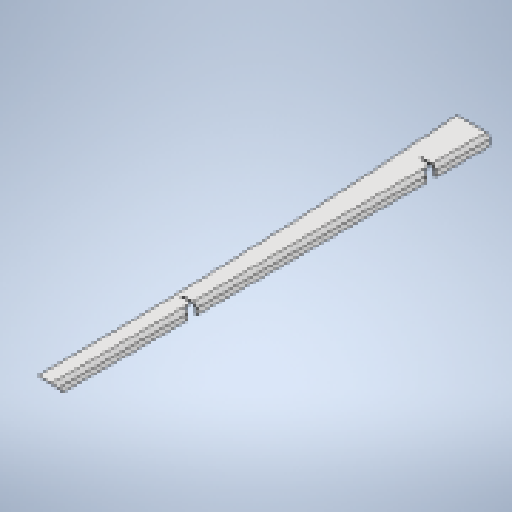
# Autodesk Inventor part: MSC 312 RIB HIP
Saved by Autodesk Inventor 2025.1 (Build 291241020, 241B)
## iProperties
Created: 2024-04-28
Part Number: MSC 312 RIB HIP
Material: Stainless Steel
Description: DIE16(5)|\ 90°|corrY -___°|X_____|bom___
Document SubType Name: Sheet Metal
Designer: pokla
Stock Number: MSC 315 шпангоут борт
Density: 8 g/cm^3
Flat Pattern Width: 91.0953 cm
Flat Pattern Length: 8.39274 cm
Flat Pattern Area: 764.54 cm^2
Sheet Metal Rule: AISI304 3mm Die 32
Sheet Metal Width: 910.953 mm
Sheet Metal Length: 83.927 mm
Sheet Metal Area: 76453.964 mm^2
Appearance: Default
Mass: 990.281 g
Surface Area: 1284.73 cm^2
Volume: 123.785 cm^3
БОРТ_стрингер_3_высота: 62,000 mm
БОРТ_стрингер_4_высота: 39,000 mm
БОРТ_стрингер_5_высота: 39,000 mm
БОРТ_стрингер_6_высота: 62,000 mm
РЕБРА_глубина_паза: 28.000 mm
РЕБРА_вырез_на_полке: 5,000 mm
РЕБРА_полка: 20,000 mm
Author: admin
Autodesk Inventor part; units mm, degrees
ref_plane "YZ Plane" through (0, 0, 0) normal (1, 0, 0) x (0, 1, 0)
ref_plane "XZ Plane" through (0, 0, 0) normal (0, 1, 0) x (-1, 0, 0)
ref_plane "XY Plane" through (0, 0, 0) normal (0, 0, 1) x (1, 0, 0)
sketch "Sketch1" plane through (0, 0, 0) normal (0, 0, 1) x (1, 0, 0)
  arc A0 (-71.9586, -1745.1712) -> (-70, 0) centre (-11089.4751, -860.2193) ccw
  line L0 (0, 0) -> (-70, 0)
  line L1 (0, -117.9106) -> (-61.4296, -117.9106) construction
  line L2 (0, -617.9106) -> (-39.1314, -617.9106) construction
  line L3 (0, -1117.9106) -> (-39.4794, -1117.9106) construction
  line L4 (0, -1617.9106) -> (-62.4758, -1617.9106) construction
  line L5 (-71.9586, -1745.1712) -> (0, -1745.1712)
  line L6 (0, 0) -> (0, -1745.1712)
  line L7 (0, -1735.1712) -> (-10.3553, -1745.1712)
  point P0 (-20, 0)
  dimension "d33" = 50
  dimension "d58" = 500
  dimension "d59" = 500
  dimension "d60" = 500
  dimension "d141" = 1745.171
  dimension "d148" = 70
  dimension "d149" = 11053
  dimension "d150" = 71.959
  dimension "d151" = 136
  dimension "d153" = 10
  measures "d33" distance of L0.end point (-20, 0)
  measures "d58" distance between parallel lines of L2 L1
  measures "d59" distance between parallel lines of L2 L3
  measures "d60" distance between parallel lines of L3 L4
  measures "d141" distance between parallel lines of L0 L5
  measures "d148" distance of L0.start L0.end
  measures "d149" radius of A0
  measures "d151" angle of L5 L7
  measures "d153" distance of L5.end L7.start
extrude "Plate3" add sketch "Sketch1" along normal blind 3 contours A0 L0 L6 L7 L5
sketch "Sketch3" plane through (-3, 0, 3) normal (1, 0, 0) x (0, 1, 0)
  line L0 (-1735.1712, 0) -> (0, 0)
  line L1 (0, 0) -> (0, 20)
  line L2 (0, 20) -> (-1735.1712, 20)
  line L3 (-1735.1712, 20) -> (-1735.1712, 0)
  constraints: 6 end point, 1 horizontal, 1 perpendicular, 1 vertical
edge flange "Flange2" height 20 angle 90 thickness 3 bend radius 5 thickness toward (1, 0, 0) relief round relief width 3 relief depth 1.5 edges at (0, -867.5856, 3) wall of the first edge with corners at (-3, -1735.1712, 3) (-3, 0, 3) (-3, 0, -17) (-3, -1735.1712, -17)
bend "Bend2"
corner "Corner2"
sketch "Sketch5" plane through (0, 0, 0) normal (0, 0, 1) x (1, 0, 0)
  line L0 (-8, -1742.8967) -> (-8, 0) projected
  line L1 (-70, 0) -> (-8, 0) projected
  arc A0 (-71.9586, -1745.1712) -> (-70, 0) centre (-11089.4751, -860.2193) ccw projected
  line L2 (0, 0) -> (0, -1735.1712) projected
  line L3 (0, -114.5) -> (-29, -114.5)
  line L4 (0, -117.5) -> (-3, -117.5) construction
  line L5 (-3, -1735.1712) -> (-3, 0) projected
  line L6 (-29, -114.5) -> (-29, -117.5)
  line L7 (0, -614.5) -> (-39.2067, -614.5) construction
  line L8 (0, -1114.5) -> (-39.4004, -1114.5) construction
  line L9 (0, -1614.5) -> (-62.242, -1614.5) construction
  line L10 (-10.3553, -1745.1712) -> (-71.9586, -1745.1712) projected
  line L11 (0, -114.5) -> (0, -134.5)
  line L12 (-3, -114.5) -> (-3, -117.5) construction
  line L13 (0, -134.5) -> (-3, -134.5)
  line L14 (-29, -114.5) -> (-61.6597, -114.5) construction
  line L15 (-29, -117.5) -> (-61.4573, -117.5) construction
  line L16 (-3, -117.5) -> (-3, -134.5)
  line L17 (-3, -117.5) -> (-29, -117.5)
  line L18 (-3, -134.5) -> (-8, -134.5)
  line L19 (-8, -1742.8967) -> (-10.3553, -1745.1712) projected
  point P0 (0, 0)
  point P1 (845.25, -380.4205)
  point P2 (848, -380.4205)
  point P3 (-29, -116)
  point P4 (850, -410.4205)
  point P5 (-3, -114.5)
  point P6 (-3, -134.5)
  point P7 (-8, -117.5)
  dimension "d69" = 1735.1712
  dimension "d70" = 3
  dimension "d76" = 61.6598
  dimension "d80" = 39.2067
  dimension "d102" = 62.242
  dimension "d104" = 39.4004
  dimension "d106" = 3
  dimension "d107" = 20
  dimension "d108" = 116
  dimension "d112" = 29
  dimension "d142" = 500
  dimension "d143" = 500
  dimension "d144" = 500
  constraints: 28 end point, 13 perpendicular, 10 point on line, 5 point on circle, 2 parallel, 1 horizontal, 1 midpoint
  measures "d69" distance of L2.start L2.end
  measures "d70" distance between parallel lines of L4 L3
  measures "d76" distance of L3.start L14.end
  measures "d80" distance of L7.start L7.end
  measures "d102" distance of L9.start L9.end
  measures "d104" distance of L8.end L8.start
  measures "d106" distance of L13.end L11.end
  measures "d107" distance of L11.end L3.start
  measures "d108" vertical distance of L2.start point (-29, -116)
  measures "d112" distance of L3.end L3.start
  measures "d142" distance between parallel lines of L7 L14
  measures "d143" distance between parallel lines of L7 L8
  measures "d144" distance between parallel lines of L9 L8
extrude "Extrusion2" cut sketch "Sketch5" along normal through all both and the other way through all contours L0 L17 L5 L18 | L17 L6 L3 L0 | L0 L3 L5 L17 | L5 L3 L2 L13
pattern_linear "Rectangular Pattern3" count 4 spacing 500 along (0, -1, 0) of "Extrusion2"
sketch "Sketch6" plane through (0, 0, 0) normal (0, 0, -1) x (-1, 0, 0)
  line L0 (25.1246, -1740.1712) -> (13.1246, -1740.1712) construction
  line L1 (13.1246, -1740.1712) -> (13.1246, -1540.1712) construction
  line L2 (13.1246, -1540.1712) -> (25.1246, -1540.1712) construction
  line L3 (25.1246, -1540.1712) -> (25.1246, -1740.1712) construction
  line L4 (25.1246, -1539.5) -> (25.1246, -1589.5) construction
  line L5 (25.1246, -1589.5) -> (13.1246, -1589.5) construction
  line L6 (13.1246, -1589.5) -> (13.1246, -1539.5) construction
  line L7 (13.1246, -1539.5) -> (25.1246, -1539.5) construction
  line L8 (8, -1614.5) -> (29, -1614.5) projected
  line L9 (25.1246, -1039.5) -> (25.1246, -1089.5) construction
  line L10 (25.1246, -1089.5) -> (13.1246, -1089.5) construction
  line L11 (13.1246, -1089.5) -> (13.1246, -1039.5) construction
  line L12 (13.1246, -1039.5) -> (25.1246, -1039.5) construction
  line L13 (25.1246, -539.5) -> (25.1246, -589.5) construction
  line L14 (25.1246, -589.5) -> (13.1246, -589.5) construction
  line L15 (13.1246, -589.5) -> (13.1246, -539.5) construction
  line L16 (13.1246, -539.5) -> (25.1246, -539.5) construction
  line L17 (25.1246, -39.5) -> (25.1246, -89.5) construction
  line L18 (25.1246, -89.5) -> (13.1246, -89.5) construction
  line L19 (13.1246, -89.5) -> (13.1246, -39.5) construction
  line L20 (13.1246, -39.5) -> (25.1246, -39.5) construction
  line L21 (8, -1114.5) -> (29, -1114.5) projected
  line L22 (8, -614.5) -> (29, -614.5) projected
  line L23 (8, -114.5) -> (29, -114.5) projected
  line L24 (25.1246, -740) -> (13.1246, -740) construction
  line L25 (13.1246, -740) -> (13.1246, -540) construction
  line L26 (13.1246, -540) -> (25.1246, -540) construction
  line L27 (25.1246, -540) -> (25.1246, -740) construction
  point P0 (0, 0)
  point P1 (71.9586, -1745.1712)
  point P2 (4.75, -1840)
  point P3 (-1.1417, -614.8288)
  point P4 (25.1083, -614.8288)
  dimension "d120" = 200
  dimension "d121" = 12
  dimension "d123" = 5
  dimension "d126" = 50
  dimension "d127" = 25
  dimension "d135" = 25
  dimension "d136" = 25
  dimension "d137" = 25
  dimension "d154" = 200
  dimension "d155" = 12
  constraints: 7 equal length, 4 collinear, 13 other
  measures "d120" distance of L0.end L1.end
  measures "d121" distance of L1.end L2.end
  measures "d126" distance of L5.end L6.end
  measures "d127" distance between parallel lines of L8 L5
  measures "d135" distance between parallel lines of L21 L10
  measures "d136" distance between parallel lines of L22 L14
  measures "d137" distance between parallel lines of L23 L18
  measures "d154" distance of L24.end L25.end
  measures "d155" distance of L25.end L26.end
chamfer "Corner Chamfer1" distance 6 angle 45 4 edges at (-8, -1617.5, 1.5) (-8, -1117.5, 1.5) (-8, -617.5, 1.5) (-8, -117.5, 1.5)
mark "Mark2"
sketch "Sketch9" plane through (0, -1614.5, -17) normal (1, 0, 0) x (0, 0, -1)
  line L0 (-17, -130.6712) -> (-20, -130.6712) projected
  line L1 (0, 500) -> (0, 980) projected
  line L2 (-20, -130.6712) -> (0, -130.6712)
  line L3 (0, -130.6712) -> (0, 720.3288)
  line L4 (0, 720.3288) -> (-20, 720.3288)
  line L5 (-20, 720.3288) -> (-20, -130.6712)
  line L6 (0, 720.3288) -> (-20, 703.5468)
  line L7 (-20, 1614.5) -> (-20, -130.6712) projected
  point P0 (-17, 1614.5)
  point P1 (-20, 703.5468)
  point P2 (0, 500)
  dimension "d163" = 851
  dimension "d164" = 40
  constraints: 10 end point, 2 parallel, 2 point on line, 1 horizontal, 1 perpendicular
  measures "d163" distance between parallel lines of L2 L4
  measures "d164" angle of L6 L4
extrude "Extrusion5" cut sketch "Sketch9" against normal through all contours L0 L5 L6 L1 L3 L2
equation "\"d33\" = d25"
equation "\"БОРТ_стрингер_3_высота\" = 62"
equation "\"БОРТ_стрингер_4_высота\" = 39"
equation "\"БОРТ_стрингер_5_высота\" = 39"
equation "\"БОРТ_стрингер_6_высота\" = 62"
equation "\"d25\" = 50"
body "Solid2"
